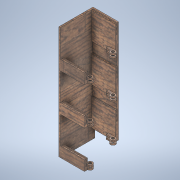
# Autodesk Inventor part: Interior Izq
Saved by Autodesk Inventor 2021 (Build 250183000, 183)
## iProperties
Created: 2021-06-27
Part Number: Interior Izq
Material: Plástico PET
Document SubType Name: Modeling
Designer: artur
Density: 1.541 g/cm^3
Appearance: Fresno blanco - Java
Mass: 608.447 g
Surface Area: 1605.23 cm^2
Volume: 394.839 cm^3
Author: artur
Autodesk Inventor part; units mm, degrees
sketch "Boceto1" plane through (0, 0, 0) normal (1, 0, 0) x (0, 1, 0)
  line L0 (0, 0) -> (330, 0)
  line L1 (330, 0) -> (330, -75)
  line L2 (330, -75) -> (0, -75)
  line L3 (0, -75) -> (0, 0)
  dimension "d0" = 75
  dimension "d1" = 330
  constraints: 8 end point, 2 parallel, 1 horizontal, 1 perpendicular
  measures "d0" distance of L0.end L1.end
  measures "d1" distance of L1.end L2.end
extrude "Extrusión1" add sketch "Boceto1" along normal blind 5
sketch "Boceto2" plane through (5, 0, 0) normal (1, 0, 0) x (0, 0, -1)
  line L0 (75, 330) -> (0, 330) construction
  line L1 (37.5, 330) -> (37.5, 250) construction
  line L2 (37.5, 250) -> (37.5, 220) construction
  line L3 (37.5, 220) -> (37.5, 140) construction
  line L4 (37.5, 140) -> (37.5, 110) construction
  line L5 (37.5, 110) -> (37.5, 30) construction
  line L6 (37.5, 30) -> (37.5, 0) construction
  line L7 (75, 0) -> (75, 330) projected
  line L8 (0, 330) -> (75, 330)
  line L9 (75, 330) -> (75, 250)
  line L10 (75, 250) -> (0, 250)
  line L11 (0, 250) -> (0, 330)
  line L12 (75, 140) -> (0, 140)
  line L13 (0, 140) -> (0, 220)
  line L14 (0, 220) -> (75, 220)
  line L15 (75, 220) -> (75, 140)
  line L16 (75, 30) -> (0, 30)
  line L17 (0, 30) -> (0, 110)
  line L18 (0, 110) -> (75, 110)
  line L19 (75, 110) -> (75, 30)
  point P0 (0, 0)
  dimension "d4" = 80
  dimension "d5" = 30
  dimension "d6" = 80
  dimension "d7" = 30
  dimension "d8" = 80
  dimension "d9" = 30
  dimension "d12" = 110
  constraints: 36 end point, 4 point on line, 4 vertical, 2 parallel, 1 horizontal, 1 midpoint, 1 perpendicular, 16 other
  measures "d4" distance of L1.start L1.end
  measures "d5" distance of L1.end L2.end
  measures "d6" distance of L2.end L3.end
  measures "d7" distance of L3.end L4.end
  measures "d8" distance of L4.end L5.end
  measures "d9" distance of L5.end L6.end
  measures "d12" distance of L9.end L12.start
extrude "Extrusión2" add sketch "Boceto2" along normal blind 4
sketch "Boceto3" plane through (0, 330, 0) normal (0, 1, 0) x (1, 0, 0)
  line L0 (7, 5) -> (4, 5)
  line L1 (4, 5) -> (4, 75)
  line L2 (4, 75) -> (7, 75)
  line L3 (7, 75) -> (7, 5)
  line L4 (0, 0) -> (9, 0) projected
  line L5 (0, 75) -> (9, 75) projected
  line L6 (9, 75) -> (9, 0) projected
  line L7 (0, 75) -> (0, 0) projected
  dimension "d22" = 5
  dimension "d23" = 0
  dimension "d24" = 2
  dimension "d73" = 3
  constraints: 8 end point, 2 parallel, 1 horizontal, 1 perpendicular
  measures "d22" distance between parallel lines of L4 L0
  measures "d23" distance between parallel lines of L5 L2
  measures "d24" distance between parallel lines of L3 L6
  measures "d73" distance between parallel lines of L1 L3
sketch "Boceto4" plane through (5, 220, 0) normal (0, 1, 0) x (1, 0, 0)
  line L0 (2, 5) -> (-1, 5) projected
  line L1 (-1, 5) -> (-1, 75) projected
  line L2 (2, 75) -> (2, 5) projected
  line L3 (-1, 75) -> (2, 75) projected
  point P0 (-5, 0)
sketch "Boceto5" plane through (5, 110, 0) normal (0, 1, 0) x (1, 0, 0)
  line L0 (2, 5) -> (-1, 5) projected
  line L1 (2, 75) -> (2, 5) projected
  line L2 (-1, 5) -> (-1, 75) projected
  line L3 (-1, 75) -> (2, 75) projected
  point P0 (-5, 0)
extrude "Extrusión3" cut sketch "Boceto3" against normal blind 30 contours L0 L1 L2 L3
extrude "Extrusión4" cut sketch "Boceto4" against normal blind 30
extrude "Extrusión5" cut sketch "Boceto5" against normal blind 30
sketch "Boceto7" plane through (0, 0, 0) normal (-1, 0, 0) x (0, 0, 1)
  line L0 (0, 0) -> (-75, 0) projected
  line L1 (-5, 330) -> (-75, 330) projected
  line L2 (0, 0) -> (-5, 0)
  line L3 (-5, 0) -> (-5, 330)
  line L4 (-5, 330) -> (0, 330)
  line L5 (0, 330) -> (0, 0)
  point P0 (-73, 330)
  dimension "d32" = 5
  constraints: 8 end point, 2 parallel, 1 horizontal, 1 perpendicular, 1 point on line
  measures "d32" distance of L3.end L4.end
extrude "Extrusión6" add sketch "Boceto7" against normal blind 100
sketch "Boceto8" plane through (9, 140, -5) normal (0, 0, -1) x (-1, 0, 0)
  line L0 (-91, -140) -> (-91, 190) projected
  line L1 (-91, 190) -> (-86, 190)
  line L2 (-86, 190) -> (-86, -140)
  line L3 (-86, -140) -> (-91, -140)
  line L4 (-91, -140) -> (-91, 190)
  point P0 (9, -140)
  dimension "d35" = 5
  dimension "d36" = 330
  constraints: 8 end point, 2 parallel, 1 horizontal, 1 perpendicular
  measures "d35" distance of L2.end L3.end
  measures "d36" distance of L1.end L2.end
extrude "Extrusión7" add sketch "Boceto8" along normal blind 70
sketch "Boceto9" plane through (95, 0, -5) normal (-1, 0, 0) x (0, 0, 1)
  line L0 (5, 330) -> (-70, 330) construction
  line L1 (-32.5, 330) -> (-32.5, 250) construction
  line L2 (-32.5, 250) -> (-32.5, 220) construction
  line L3 (-32.5, 220) -> (-32.5, 140) construction
  line L4 (-32.5, 140) -> (-32.5, 110) construction
  line L5 (-32.5, 110) -> (-32.5, 30) construction
  line L6 (-32.5, 30) -> (-32.5, 0) construction
  line L7 (5, 0) -> (-70, 0) construction
  line L8 (0, 330) -> (0, 0) projected
  line L9 (0, 220) -> (-70, 220)
  line L10 (-70, 220) -> (-70, 250)
  line L11 (-70, 250) -> (0, 250)
  line L12 (0, 250) -> (0, 220)
  line L13 (-70, 140) -> (0, 140)
  line L14 (-70, 110) -> (-70, 140)
  line L15 (0, 110) -> (-70, 110)
  line L16 (0, 140) -> (0, 110)
  line L17 (-70, 30) -> (0, 30)
  line L18 (-70, 0) -> (-70, 30)
  line L19 (0, 0) -> (-70, 0)
  line L20 (0, 30) -> (0, 0)
  line L21 (-70, -80) -> (0, -80)
  line L22 (-70, -110) -> (-70, -80)
  line L23 (0, -110) -> (-70, -110)
  line L24 (0, -80) -> (0, -110)
  line L25 (-70, -190) -> (0, -190)
  line L26 (-70, -220) -> (-70, -190)
  line L27 (0, -220) -> (-70, -220)
  line L28 (0, -190) -> (0, -220)
  line L29 (-70, -300) -> (0, -300)
  line L30 (-70, -330) -> (-70, -300)
  line L31 (0, -330) -> (-70, -330)
  line L32 (0, -300) -> (0, -330)
  line L33 (-70, -410) -> (0, -410)
  line L34 (-70, -440) -> (-70, -410)
  line L35 (0, -440) -> (-70, -440)
  line L36 (0, -410) -> (0, -440)
  line L37 (-70, -520) -> (0, -520)
  line L38 (-70, -550) -> (-70, -520)
  line L39 (0, -550) -> (-70, -550)
  line L40 (0, -520) -> (0, -550)
  line L41 (-70, -630) -> (0, -630)
  line L42 (-70, -660) -> (-70, -630)
  line L43 (0, -660) -> (-70, -660)
  line L44 (0, -630) -> (0, -660)
  line L45 (-70, -740) -> (0, -740)
  line L46 (-70, -770) -> (-70, -740)
  line L47 (0, -770) -> (-70, -770)
  line L48 (0, -740) -> (0, -770)
  line L49 (-70, -850) -> (0, -850)
  line L50 (-70, -880) -> (-70, -850)
  line L51 (0, -880) -> (-70, -880)
  line L52 (0, -850) -> (0, -880)
  line L53 (-70, -960) -> (0, -960)
  line L54 (-70, -990) -> (-70, -960)
  line L55 (0, -990) -> (-70, -990)
  line L56 (0, -960) -> (0, -990)
  line L57 (-70, -1070) -> (0, -1070)
  line L58 (-70, -1100) -> (-70, -1070)
  line L59 (0, -1100) -> (-70, -1100)
  line L60 (0, -1070) -> (0, -1100)
  line L61 (-70, -1180) -> (0, -1180)
  line L62 (-70, -1210) -> (-70, -1180)
  line L63 (0, -1210) -> (-70, -1210)
  line L64 (0, -1180) -> (0, -1210)
  line L65 (-70, -1290) -> (0, -1290)
  line L66 (-70, -1320) -> (-70, -1290)
  line L67 (0, -1320) -> (-70, -1320)
  line L68 (0, -1290) -> (0, -1320)
  line L69 (-70, -1400) -> (0, -1400)
  line L70 (-70, -1430) -> (-70, -1400)
  line L71 (0, -1430) -> (-70, -1430)
  line L72 (0, -1400) -> (0, -1430)
  line L73 (-70, -1510) -> (0, -1510)
  line L74 (-70, -1540) -> (-70, -1510)
  line L75 (0, -1540) -> (-70, -1540)
  line L76 (0, -1510) -> (0, -1540)
  line L77 (-70, -1620) -> (0, -1620)
  line L78 (-70, -1650) -> (-70, -1620)
  line L79 (0, -1650) -> (-70, -1650)
  line L80 (0, -1620) -> (0, -1650)
  line L81 (-70, -1730) -> (0, -1730)
  line L82 (-70, -1760) -> (-70, -1730)
  line L83 (0, -1760) -> (-70, -1760)
  line L84 (0, -1730) -> (0, -1760)
  line L85 (-70, -1840) -> (0, -1840)
  line L86 (-70, -1870) -> (-70, -1840)
  line L87 (0, -1870) -> (-70, -1870)
  line L88 (0, -1840) -> (0, -1870)
  line L89 (-70, -1950) -> (0, -1950)
  line L90 (-70, -1980) -> (-70, -1950)
  line L91 (0, -1980) -> (-70, -1980)
  line L92 (0, -1950) -> (0, -1980)
  line L93 (-70, -2060) -> (0, -2060)
  line L94 (-70, -2090) -> (-70, -2060)
  line L95 (0, -2090) -> (-70, -2090)
  line L96 (0, -2060) -> (0, -2090)
  line L97 (-70, -2170) -> (0, -2170)
  line L98 (-70, -2200) -> (-70, -2170)
  line L99 (0, -2200) -> (-70, -2200)
  line L100 (0, -2170) -> (0, -2200)
  line L101 (-70, -2280) -> (0, -2280)
  line L102 (-70, -2310) -> (-70, -2280)
  line L103 (0, -2310) -> (-70, -2310)
  line L104 (0, -2280) -> (0, -2310)
  line L105 (-70, -2390) -> (0, -2390)
  line L106 (-70, -2420) -> (-70, -2390)
  line L107 (0, -2420) -> (-70, -2420)
  line L108 (0, -2390) -> (0, -2420)
  line L109 (-70, -2500) -> (0, -2500)
  line L110 (-70, -2530) -> (-70, -2500)
  line L111 (0, -2530) -> (-70, -2530)
  line L112 (0, -2500) -> (0, -2530)
  line L113 (-70, -2610) -> (0, -2610)
  line L114 (-70, -2640) -> (-70, -2610)
  line L115 (0, -2640) -> (-70, -2640)
  line L116 (0, -2610) -> (0, -2640)
  line L117 (-70, -2720) -> (0, -2720)
  line L118 (-70, -2750) -> (-70, -2720)
  line L119 (0, -2750) -> (-70, -2750)
  line L120 (0, -2720) -> (0, -2750)
  line L121 (-70, -2830) -> (0, -2830)
  line L122 (-70, -2860) -> (-70, -2830)
  line L123 (0, -2860) -> (-70, -2860)
  line L124 (0, -2830) -> (0, -2860)
  line L125 (-70, -2940) -> (0, -2940)
  line L126 (-70, -2970) -> (-70, -2940)
  line L127 (0, -2970) -> (-70, -2970)
  line L128 (0, -2940) -> (0, -2970)
  point P0 (0, 0)
  dimension "d39" = 80
  dimension "d40" = 30
  dimension "d41" = 80
  dimension "d42" = 30
  dimension "d43" = 80
  dimension "d46" = 110
  constraints: 252 end point, 5 point on line, 2 midpoint, 2 parallel, 2 vertical, 1 horizontal, 1 perpendicular, 232 other
  measures "d39" distance of L1.start L1.end
  measures "d40" distance of L1.end L2.end
  measures "d41" distance of L2.end L3.end
  measures "d42" distance of L3.end L4.end
  measures "d43" distance of L4.end L5.end
  measures "d46" distance of L10.end L13.start
extrude "Extrusión8" add sketch "Boceto9" along normal blind 4 contours L8 L19 L18 L17 | L8 L15 L14 L13 | L8 L9 L10 L11
sketch "Boceto14" plane through (100, 0, 0) normal (1, 0, 0) x (0, 0, -1)
  line L0 (75, 140) -> (5, 140) projected
  line L1 (5, 220) -> (5, 140) projected
  line L2 (5, 220) -> (75, 220) projected
  line L3 (75, 140) -> (75, 220) projected
  line L4 (75, 30) -> (5, 30) projected
  line L5 (5, 110) -> (5, 30) projected
  line L6 (5, 110) -> (75, 110) projected
  line L7 (75, 30) -> (75, 110) projected
  line L8 (75, 250) -> (5, 250) projected
  line L9 (5, 330) -> (5, 250) projected
  line L10 (5, 330) -> (75, 330) projected
  line L11 (75, 250) -> (75, 330) projected
  point P0 (0, 0)
extrude "Extrusión13" cut sketch "Boceto14" against normal blind 10
sketch "Boceto15" plane through (0, 0, -75) normal (0, 0, -1) x (-1, 0, 0)
  line L0 (-7, 300) -> (-7, 330) projected
  line L1 (-7, 330) -> (-9, 328.1395)
  line L2 (-7, 330) -> (-5.0608, 330) construction
  line L3 (-9, 250) -> (-9, 330) projected
  line L4 (-9, 328.1395) -> (-9, 330)
  line L5 (-9, 330) -> (-7, 330)
  line L6 (0, 330) -> (-100, 330) projected
  line L7 (-7, 220) -> (-9, 218.1395)
  line L8 (-9, 140) -> (-9, 220) projected
  line L9 (-7, 220) -> (-9, 220) projected
  line L10 (-9, 220) -> (-7, 220)
  line L11 (-7, 80) -> (-7, 110) projected
  line L12 (-7, 110) -> (-8.4215, 108.6777)
  line L13 (-7, 110) -> (-5.0585, 110) construction
  line L14 (-7, 110) -> (-9, 110) projected
  line L15 (-7, 110) -> (-9, 110)
  line L16 (-9, 110) -> (-9, 108.1395)
  line L17 (-9, 30) -> (-9, 110) projected
  point P0 (0, 0)
  dimension "d183" = 42.93
  dimension "d184" = 42.93
  dimension "d185" = 42.93
  constraints: 20 end point, 5 point on line, 4 horizontal, 1 collinear, 1 equal length
  measures "d183" angle of L5 L1
  measures "d184" angle of L14 L12
  measures "d185" angle of L9 L7
extrude "Extrusión14" cut sketch "Boceto15" against normal blind 70
sketch "Boceto16" plane through (5, 0, 0) normal (1, 0, 0) x (0, 0, -1)
  line L0 (5, 0) -> (75, 0) projected
  line L1 (75, 0) -> (75, 30) projected
  line L2 (75, 30) -> (5, 30) projected
  line L3 (5, 30) -> (5, 0) projected
  point P0 (0, 0)
extrude "Extrusión15" cut sketch "Boceto16" against normal blind 10
sketch "Boceto17" plane through (91, 220, -5) normal (0, -1, 0) x (1, 0, 0)
  line L0 (0, -69.9614) -> (-43.9191, -69.9614) construction
  circle A0 centre (-7.5, -69.9614) radius 7.5
  line L1 (0, -49.9614) -> (-7.5, -49.9614)
  line L2 (-7.5, -49.9614) -> (-7.5, -69.9614)
  line L3 (-7.5, -69.9614) -> (0, -69.9614)
  line L4 (0, -69.9614) -> (0, -49.9614)
  circle A1 centre (-7.5, -69.9614) radius 4
  line L5 (0, -70) -> (0, 0) projected
  point P0 (-91, 5)
  point P1 (-7.5, -62.4614)
  point P2 (0, -69.9614)
  dimension "d81" = 15
  dimension "d80" = 20
  dimension "d82" = 8
  dimension "d83" = 7.5
  dimension "d84" = 0
  constraints: 10 end point, 2 horizontal, 2 parallel, 1 centre point, 1 coincident, 1 perpendicular, 1 point on line, 3 other
  measures "d80" distance of L1.end L2.end
  measures "d82" diameter of A1
  measures "d83" distance of L2.end L3.end
  measures "d84" distance between parallel lines of L5 L4
sketch "Boceto18" plane through (91, 110, -5) normal (0, -1, 0) x (1, 0, 0)
  line L0 (0, -69.9614) -> (0, -49.9614) projected
  line L1 (0, -49.9614) -> (-7.5, -49.9614) projected
  line L2 (-7.5, -49.9614) -> (-7.5, -69.9614) projected
  line L3 (-7.5, -69.9614) -> (0, -69.9614) projected
  circle A0 centre (-7.5, -69.9614) radius 7.5 projected
  circle A1 centre (-7.5, -69.9614) radius 4 projected
  point P0 (-91, 5)
  point P1 (-7.5, -62.4614)
sketch "Boceto19" plane through (0, 0, -5) normal (0, -1, 0) x (1, 0, 0)
  line L0 (91, -69.9614) -> (91, -49.9614) projected
  line L1 (83.5, -69.9614) -> (91, -69.9614) projected
  line L2 (91, -49.9614) -> (83.5, -49.9614) projected
  line L3 (83.5, -49.9614) -> (83.5, -69.9614) projected
  circle A0 centre (83.5, -69.9614) radius 4 projected
  circle A1 centre (83.5, -69.9614) radius 7.5 projected
  point P0 (0, 5)
  point P1 (91, -69.9614)
  point P2 (83.5, -62.4614)
extrude "Extrusión16" add sketch "Boceto19" against normal blind 12.6 contours A1 L3 L2 L0 | A1 L3 A0 L1 | L1 A0 L3 A1
extrude "Extrusión17" add sketch "Boceto18" against normal blind 12.6 contours A0 L2 L1 L0 | A0 L2 A1 L3 | L3 A1 L2 A0
extrude "Extrusión18" add sketch "Boceto17" against normal blind 12.6 contours A0 L2 A1 L3 | L3 A1 L2 A0 | A0 L2 L1 L4
ref_plane "Plano de trabajo1" through (0, 6.3, -5) normal (0, 1, 0) x (1, 0, 0)
ref_plane "Plano de trabajo2" through (91, 116.3, -5) normal (0, 1, 0) x (1, 0, 0)
ref_plane "Plano de trabajo3" through (91, 226.3, -5) normal (0, 1, 0) x (1, 0, 0)
sketch "Boceto20" plane through (0, 6.3, -5) normal (0, 1, 0) x (1, 0, 0)
  circle A0 centre (83.5, 69.9614) radius 4 projected
  line L0 (0, 0) -> (91, 0) projected
  line L1 (91, 49.9614) -> (91, 0) projected
  line L2 (91, 49.9614) -> (83.5, 49.9614) projected
  line L3 (83.5, 49.9614) -> (83.5, 62.4614) projected
  arc A1 (91, 69.9614) -> (83.5, 62.4614) centre (83.5, 69.9614) ccw projected
  line L4 (91, 70) -> (91, 69.9614) projected
  line L5 (100, 70) -> (91, 70) projected
  line L6 (100, -5) -> (100, 70) projected
  line L7 (0, -5) -> (100, -5) projected
  line L8 (0, -5) -> (0, 0) projected
  line L9 (91, 0) -> (91, 70) projected
  line L10 (91, 49.9614) -> (91, 70)
  point P0 (91, 69.9614)
  point P1 (91, 69.9614)
  constraints: 2 end point
extrude "Extrusión19" cut sketch "Boceto20" along normal mid plane 4.2 contours L2 L3 A1 L9
sketch "Boceto22" plane through (91, 226.3, -5) normal (0, 1, 0) x (1, 0, 0)
  circle A0 centre (-7.5, 69.9614) radius 4 projected
  line L0 (9, 0) -> (0, 0) projected
  line L1 (0, 49.9614) -> (0, 0) projected
  line L2 (0, 49.9614) -> (-7.5, 49.9614) projected
  line L3 (-7.5, 49.9614) -> (-7.5, 62.4614) projected
  arc A1 (0, 69.9614) -> (-7.5, 62.4614) centre (-7.5, 69.9614) ccw projected
  line L4 (0, 70) -> (0, 69.9614) projected
  line L5 (9, 70) -> (0, 70) projected
  line L6 (9, 0) -> (9, 70) projected
  line L7 (-7.5, 49.9614) -> (0, 49.9614) projected
  line L8 (0, 49.9614) -> (0, 70)
  point P0 (-91, -5)
  constraints: 2 end point, 1 perpendicular
extrude "Extrusión21" cut sketch "Boceto22" along normal mid plane 4.2 contours L2 L3 A1 L8
sketch "Boceto23" plane through (91, 116.3, -5) normal (0, 1, 0) x (1, 0, 0)
  circle A0 centre (-7.5, 69.9614) radius 4 projected
  line L0 (-91, 0) -> (0, 0) projected
  line L1 (0, 49.9614) -> (0, 0) projected
  line L2 (0, 49.9614) -> (-7.5, 49.9614) projected
  line L3 (-7.5, 49.9614) -> (-7.5, 62.4614) projected
  arc A1 (0, 69.9614) -> (-7.5, 62.4614) centre (-7.5, 69.9614) ccw projected
  line L4 (0, 70) -> (0, 69.9614) projected
  line L5 (9, 70) -> (0, 70) projected
  line L6 (9, -5) -> (9, 70) projected
  line L7 (-91, -5) -> (9, -5) projected
  line L8 (-91, -5) -> (-91, 0) projected
  line L9 (0, 0) -> (0, 70) projected
  line L10 (0, 49.9614) -> (0, 70)
  constraints: 2 end point, 1 collinear
extrude "Extrusión22" cut sketch "Boceto23" against normal mid plane 4.2 contours L2 L3 A1 L9
thread "Rosca1" size "M8x1.25" class "6H" standard "ANSI Metric M Profile" full length
sketch "Sketch24" plane through (5, 250, -75) normal (0, -1, 0) x (1, 0, 0)
  line L0 (4, 75) -> (4, 0) projected
  line L1 (4, 0) -> (4, 20)
  line L2 (4, 20) -> (11.5, 20)
  line L3 (11.5, 20) -> (11.5, 0)
  line L4 (11.5, 0) -> (4, 0)
  circle A0 centre (11.5, 0) radius 4
  circle A1 centre (11.5, 0) radius 7.5
  point P0 (-5, 75)
  point P1 (4, 70)
  point P2 (11.5, 7.5)
  dimension "d102" = 20
  dimension "d103" = 7.5
  dimension "d140" = 8
  dimension "d141" = 15
  constraints: 8 end point, 3 perpendicular, 2 centre point, 2 coincident, 1 point on line
  measures "d102" distance of L0.end L1.end
  measures "d103" distance of L1.end L2.end
  measures "d140" diameter of A0
  measures "d141" diameter of A1
extrude "Extrusion30" add sketch "Sketch24" against normal blind 12.6 contours L2 L3 A1 L0 | A1 L3 A0 L4 | L4 A0 L3 A1
ref_plane "Work Plane8" through (5, 256.3, -75) normal (0, 1, 0) x (1, 0, 0)
sketch "Sketch30" plane through (5, 256.3, -75) normal (0, 1, 0) x (1, 0, 0)
  line L0 (11.5, -20) -> (4, -20)
  line L1 (4, -20) -> (4, 0)
  line L2 (4, 0) -> (11.5, 0)
  line L3 (11.5, 0) -> (11.5, -20)
  circle A0 centre (11.5, 0) radius 4
  circle A1 centre (11.5, 0) radius 7.5
  point P0 (-5, -75)
  point P1 (11.5, -7.5)
  point P2 (7.5, 0)
  point P3 (11.5, -4)
  dimension "d147" = 7.5
  dimension "d148" = 20
  dimension "d149" = 8
  dimension "d150" = 15
  constraints: 8 end point, 3 perpendicular, 2 centre point, 2 coincident, 1 horizontal
  measures "d147" distance of L0.start L0.end
  measures "d148" distance of L0.end L1.end
  measures "d149" diameter of A0
  measures "d150" diameter of A1
extrude "Extrusion31" cut sketch "Sketch30" against normal mid plane 4.2 contours L0 L1 A1 L3 | A1 L2 A0 L3 | L3 A0 L2 A1 | A0 L2 L3 picked at (9.6262, -1.8738)
sketch "Sketch31" plane through (5, 140, -75) normal (0, -1, 0) x (1, 0, 0)
  line L0 (0, 0) -> (4, 0) projected
  line L1 (4, 0) -> (4, 20)
  line L2 (4, 70) -> (4, 0) projected
  line L3 (4, 20) -> (11.5, 20)
  line L4 (11.5, 20) -> (11.5, 0)
  line L5 (11.5, 0) -> (4, 0)
  circle A0 centre (11.5, 0) radius 4
  circle A1 centre (11.5, 0) radius 7.5
  point P0 (-5, 75)
  point P1 (11.5, 7.5)
  dimension "d153" = 20
  dimension "d154" = 7.5
  dimension "d155" = 8
  dimension "d156" = 15
  constraints: 8 end point, 2 centre point, 2 coincident, 2 perpendicular, 1 collinear, 1 point on line
  measures "d153" distance of L0.end L1.end
  measures "d154" distance of L1.end L3.end
  measures "d155" diameter of A0
  measures "d156" diameter of A1
extrude "Extrusion32" add sketch "Sketch31" against normal blind 12.6 contours A1 L4 A0 L5 | L5 A0 L4 A1 | L1 L3 L4 A1
ref_plane "Work Plane9" through (5, 146.3, -75) normal (0, -1, 0) x (1, 0, 0)
sketch "Sketch32" plane through (5, 146.3, -75) normal (0, -1, 0) x (1, 0, 0)
  line L0 (11.5, 20) -> (11.5, 0)
  line L1 (11.5, 0) -> (4, 0)
  line L2 (4, 0) -> (4, 20)
  line L3 (4, 20) -> (11.5, 20)
  circle A0 centre (11.5, 0) radius 4
  circle A1 centre (11.5, 0) radius 7.5
  point P0 (-5, 75)
  point P1 (11.5, 7.5)
  dimension "d160" = 20
  dimension "d161" = 7.5
  dimension "d162" = 20
  dimension "d163" = 8
  dimension "d164" = 15
  constraints: 8 end point, 2 centre point, 2 coincident, 1 perpendicular, 1 vertical
  measures "d160" distance of L0.start L0.end
  measures "d161" distance of L0.end L1.end
  measures "d162" distance of L1.end L2.end
  measures "d163" diameter of A0
  measures "d164" diameter of A1
extrude "Extrusion33" cut sketch "Sketch32" against normal mid plane 4.2 contours L0 A1 L2 L3 | A1 L1 A0 L0 | L0 A0 L1 A1
sketch "Sketch33" plane through (0, 30, -75) normal (0, -1, 0) x (1, 0, 0)
  line L0 (9, 0) -> (9, 20)
  line L1 (9, 20) -> (16.5, 20)
  line L2 (16.5, 20) -> (16.5, 0)
  line L3 (16.5, 0) -> (9, 0)
  circle A0 centre (16.5, 0) radius 4
  circle A1 centre (16.5, 0) radius 7.5
  point P0 (0, 75)
  point P1 (16.5, 7.5)
  dimension "d167" = 20
  dimension "d168" = 7.5
  dimension "d169" = 8
  dimension "d170" = 15
  constraints: 8 end point, 3 perpendicular, 2 centre point, 2 coincident, 1 vertical
  measures "d167" distance of L0.start L0.end
  measures "d168" distance of L0.end L1.end
  measures "d169" diameter of A0
  measures "d170" diameter of A1
extrude "Extrusion34" add sketch "Sketch33" against normal blind 12.6 contours A1 L2 A0 L3 | L3 A0 L2 A1 | L0 L1 L2 A1
ref_plane "Work Plane10" through (0, 36.3, -5) normal (0, -1, 0) x (1, 0, 0)
sketch "Sketch34" plane through (0, 36.3, -5) normal (0, -1, 0) x (1, 0, 0)
  circle A0 centre (16.5, -70) radius 4 projected
  line L0 (16.5, -50) -> (16.5, -70)
  line L1 (16.5, -70) -> (9, -70)
  line L2 (9, -70) -> (9, -50)
  line L3 (9, -50) -> (16.5, -50)
  circle A1 centre (16.5, -70) radius 4
  circle A2 centre (16.5, -70) radius 7.5
  point P0 (0, 5)
  point P1 (16.5, -62.5)
  dimension "d174" = 20
  dimension "d175" = 7.5
  dimension "d176" = 20
  dimension "d177" = 8
  dimension "d178" = 15
  constraints: 8 end point, 2 centre point, 2 coincident, 2 perpendicular, 1 vertical
  measures "d174" distance of L0.start L0.end
  measures "d175" distance of L0.end L1.end
  measures "d176" distance of L1.end L2.end
  measures "d177" diameter of A1
  measures "d178" diameter of A2
extrude "Extrusion35" cut sketch "Sketch34" along normal mid plane 4.2 contours A0 L0 A2 L1 | A0 L1 A2 L0 | A2 L2 L3 L0
thread "Thread3" size "M8x1.25" class "6H" standard "ANSI Metric M Profile" full length
sketch "Boceto10" plane through (95, 250, -5) normal (0, 1, 0) x (1, 0, 0)
  line L0 (5, 0) -> (-4, 0) projected
  line L1 (5, 70) -> (-4, 70) projected
  line L2 (-2, 0) -> (1, 0)
  line L3 (1, 0) -> (1, 70)
  line L4 (1, 70) -> (-2, 70)
  line L5 (-2, 70) -> (-2, 0)
  line L6 (-4, 0) -> (-4, 70) projected
  point P0 (-2, 70)
  point P1 (1, 0)
  dimension "d192" = 2
  dimension "d193" = 3
  constraints: 8 end point, 2 parallel, 2 point on line, 1 horizontal, 1 perpendicular
  measures "d192" distance between parallel lines of L5 L6
  measures "d193" distance between parallel lines of L5 L3
extrude "Extrusión36" cut sketch "Boceto10" against normal blind 20 contours L0 L5 L1 L3
pattern_linear "Patrón rectangular1" count 3 spacing 110 along (0, -1, 0) of "Extrusión36"
equation "\"d184\" = d183"
equation "\"d185\" = d183"
